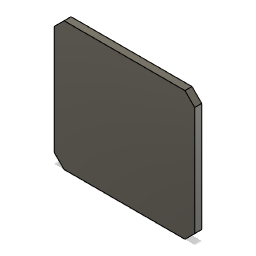
Hero7 Mask (Autodesk Fusion 360 archive; units mm, degrees)
design "ND-Filter_TBS"
Autodesk Fusion 360 part; units mm, degrees
sketch "Skizze1" plane through (0, 0, 0) normal (0, 0, 1) x (1, 0, 0)
  line L0 (18, 16.5) -> (-18, 16.5)
  line L1 (-18, 16.5) -> (-18, -16.5)
  line L2 (-18, -16.5) -> (18, -16.5)
  line L3 (18, -16.5) -> (18, 16.5)
  line L4 (18, 14) -> (15.5, 16.5)
  line L5 (-15.5, 16.5) -> (-18, 14)
  line L6 (18, -14) -> (15.5, -16.5)
  line L7 (-18, -14) -> (-15.5, -16.5)
  dimension "d1" = 36
  dimension "d2" = 33
  dimension "d3" = 18
  dimension "d4" = 16.5
  dimension "d5" = 2.5
  dimension "d6" = 45
  dimension "d7" = 45
  dimension "d8" = 2.5
  dimension "d9" = 45
  constraint horizontal L0
  constraint vertical L1
  constraint horizontal L2
  constraint vertical L3
  constraint coincident L3 L4.start
  constraint coincident L0 L4.end
  constraint coincident L0 L5.start
  constraint coincident L1 L5.end
  constraint coincident L3 L6.start
  constraint coincident L2 L6.end
  constraint parallel L5 L6
  constraint coincident L1 L7.start
  constraint coincident L2 L7.end
  constraint parallel L4 L7
  constraint vertical L4.end L6.end
  constraint vertical L5.start L7.end
  measures "d1" distance of L0.start L0.end
  measures "d2" distance of L0.end L1.end
  measures "d3" distance of origin L1
  measures "d4" distance of origin L0
  measures "d5" distance of L3 L4.end
  measures "d6" angle of L0 L4
  measures "d7" angle of L0 L5
  measures "d8" distance of L1 L5.start
  measures "d9" angle of L2 L6
extrude "Extrusion1" add sketch "Skizze1" along normal blind 1.8 contours L0 L1 L2 L3 L4 L5 L6 L7
equation "d3 = d1 / 2"
equation "d4 = d2 / 2"
equation "d8 = d5"
